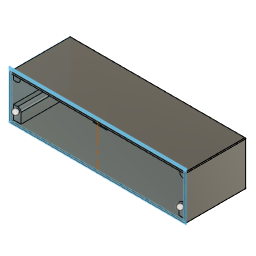
Midi Thru Box Enclosure v1 (Autodesk Fusion 360 design; units mm, degrees)
Autodesk Fusion 360 part; units mm, degrees
sketch "Sketch1" plane through (0, 0, 0) normal (0, 1, 0) x (1, 0, 0)
  line L0 (-3.1741, -17.9194) -> (125.8259, -17.9194) construction
  line L1 (125.8259, -17.9194) -> (125.8259, 15.0806) construction
  line L2 (125.8259, 15.0806) -> (-3.1741, 15.0806) construction
  line L3 (-3.1741, 15.0806) -> (-3.1741, -17.9194) construction
  circle A0 centre (-0.1741, 7.5806) radius 1.5 construction
  line L4 (61.3259, -17.9194) -> (61.3259, 15.0806)
  circle A1 centre (122.8259, 7.5806) radius 1.5 construction
  line L5 (-3.2741, -18.0194) -> (125.9259, -18.0194)
  line L6 (125.9259, -18.0194) -> (125.9259, 15.1806)
  line L7 (125.9259, 15.1806) -> (-3.2741, 15.1806)
  line L8 (-3.2741, 15.1806) -> (-3.2741, -18.0194)
  line L9 (-4.4741, -19.2194) -> (127.1259, -19.2194)
  line L10 (127.1259, -19.2194) -> (127.1259, 16.3806)
  line L11 (127.1259, 16.3806) -> (-4.4741, 16.3806)
  line L12 (-4.4741, 16.3806) -> (-4.4741, -19.2194)
  dimension "d1" = 129
  dimension "d2" = 33
  dimension "d6" = 3
  dimension "d7" = 6
  dimension "d8" = 1.5
  dimension "d11" = 0.1
  dimension "d12" = 1.3
  constraint horizontal L0
  constraint vertical L1
  constraint horizontal L2
  constraint vertical L3
  constraint midpoint L0 L4.start
  constraint midpoint L2 L4.end
  constraint symmetric A0 L4 A1
  measures "d1" distance of L0.start L0.end
  measures "d2" distance of L0.start L2.end
  measures "d6" diameter of A0
  measures "d7" distance of L2 A0
  measures "d8" distance of L3 A0
extrude "Extrude1" add sketch "Sketch1" along normal blind 44 makes body 1
sketch "Sketch2" plane through (0, 44, 0) normal (0, 1, 0) x (-1, 0, 0)
  line L0 (3.2741, 18.0194) -> (3.2741, -15.1806)
  line L1 (3.2741, -15.1806) -> (-125.9259, -15.1806)
  line L2 (-125.9259, -15.1806) -> (-125.9259, 18.0194)
  line L3 (-125.9259, 18.0194) -> (3.2741, 18.0194)
  line L4 (4.4741, -16.3806) -> (4.4741, 19.2194)
  line L5 (4.4741, 19.2194) -> (-127.1259, 19.2194)
  line L6 (-127.1259, 19.2194) -> (-127.1259, -16.3806)
  line L7 (-127.1259, -16.3806) -> (4.4741, -16.3806)
extrude "Extrude2" add sketch "Sketch2" along normal blind 1.2 contours L0 L1 L2 L3 | L4 L5 L6 L7 bodies 1
sketch "Sketch3" plane through (-3.2741, 0, 0) normal (1, 0, 0) x (0, 1, 0)
  line L0 (0, 18.0194) -> (0, -15.1806)
  line L1 (0, -15.1806) -> (44, -15.1806)
  line L2 (44, -15.1806) -> (44, 18.0194)
  line L3 (44, 18.0194) -> (0, 18.0194)
sketch "Sketch4" plane through (0, 44, 0) normal (0, -1, 0) x (1, 0, 0)
  line L0 (125.9259, 18.0194) -> (-3.2741, 18.0194)
  line L1 (-3.2741, 18.0194) -> (-3.2741, -15.1806)
  line L2 (-3.2741, -15.1806) -> (125.9259, -15.1806)
  line L3 (125.9259, -15.1806) -> (125.9259, 18.0194)
  line L4 (-3.2741, 18.0194) -> (1.7259, 18.0194)
  line L5 (1.7259, 18.0194) -> (1.7259, 15.5194)
  line L6 (-0.7741, 13.0194) -> (-3.2741, 13.0194)
  line L7 (-3.2741, 13.0194) -> (-3.2741, 18.0194)
  arc A0 (-0.7741, 13.0194) -> (1.7259, 15.5194) centre (-0.7741, 15.5194) ccw
  line L8 (61.3259, 18.0194) -> (61.3259, -15.1806)
  line L9 (-3.2741, 1.4194) -> (125.9259, 1.4194)
  line L10 (120.9259, 18.0194) -> (120.9259, 15.5194)
  line L11 (125.9259, 18.0194) -> (120.9259, 18.0194)
  line L12 (125.9259, 13.0194) -> (125.9259, 18.0194)
  line L13 (123.4259, 13.0194) -> (125.9259, 13.0194)
  arc A1 (120.9259, 15.5194) -> (123.4259, 13.0194) centre (123.4259, 15.5194) ccw
  line L14 (-3.2741, -15.1806) -> (2.7259, -15.1806)
  line L15 (-3.2741, -4.6806) -> (-3.2741, -15.1806)
  circle A2 centre (-0.1741, -7.5806) radius 1.5
  circle A3 centre (-0.1741, -7.5806) radius 1.3
  line L16 (-3.2741, -5.0806) -> (-0.1741, -5.0806)
  line L17 (2.3259, -7.5806) -> (2.3259, -15.1806)
  arc A4 (2.3259, -7.5806) -> (-0.1741, -5.0806) centre (-0.1741, -7.5806) ccw
  line L18 (61.3259, 17.9194) -> (61.3259, -15.0806)
  line L19 (125.9259, -5.0806) -> (122.8259, -5.0806)
  arc A5 (122.8259, -5.0806) -> (120.3259, -7.5806) centre (122.8259, -7.5806) ccw
  line L20 (120.3259, -7.5806) -> (120.3259, -15.1806)
  circle A6 centre (122.8259, -7.5806) radius 1.3
  dimension "d17" = 5
  dimension "d18" = 5
  dimension "d19" = 2.5
  dimension "d24" = 2.6
  dimension "d25" = 5
  constraint horizontal L4
  constraint vertical L5
  constraint horizontal L6
  constraint vertical L7
  constraint coincident L0.end L1.start
  constraint tangent L5 A0
  constraint tangent L6 A0
  constraint midpoint L0 L8.start
  constraint midpoint L2 L8.end
  constraint midpoint L1 L9.start
  constraint midpoint L3 L9.end
  constraint symmetric L0.end L8 L0.start
  constraint symmetric L4.end L8 L10.start
  constraint symmetric L6.end L8 L12.start
  constraint symmetric L5.end L8 L10.end
  constraint symmetric L6.start L8 L13.start
  constraint symmetric A0 L8 A1
  constraint horizontal L14
  constraint vertical L15
  constraint coincident L1.end L2.start
  constraint concentric A2 A3
  constraint concentric A3 A4
  constraint coincident L15 L16.start
  constraint horizontal L16
  constraint tangent L16 A4
  constraint coincident L2 L17.end
  constraint perpendicular L2 L17
  constraint tangent L17 A4
  constraint symmetric A3 L18 A6
  constraint symmetric L16.start L18 L19.start
  constraint symmetric L17.end L18 L20.end
  constraint symmetric L16.end L18 L19.end
  constraint symmetric L17.start L18 A5.end
  constraint symmetric A4 L18 A5
  measures "d17" distance of L0.end L4.end
  measures "d18" distance of L0.end L6.end
  measures "d19" radius of A0
  measures "d24" diameter of A3
  measures "d25" diameter of A4
extrude "Extrude3" add sketch "Sketch4" along normal blind 42.3 contours L0 L3 L10 L11 L12 L13 A1 | L0 L1 L4 L5 L6 L7 A0 | L2 L3 L19 A5 L20 | L1 L2 L14 L15 L16 L17 A4 | A2 | A3 | A6 bodies 1
sketch "Sketch5" plane through (0, 1.7, 0) normal (0, -1, 0) x (1, 0, 0)
  line L0 (-3.2741, -5.0806) -> (-3.2741, -15.1806)
  line L1 (-3.2741, -15.1806) -> (2.3259, -15.1806)
  line L2 (2.3259, -15.1806) -> (2.3259, -7.5806)
  arc A0 (2.3259, -7.5806) -> (-0.1741, -5.0806) centre (-0.1741, -7.5806) ccw
  line L3 (-0.1741, -5.0806) -> (-3.2741, -5.0806)
  circle A1 centre (-0.1741, -7.5806) radius 1.5
  circle A2 centre (-0.1741, -7.5806) radius 1.3
  circle A3 centre (122.8259, -7.5806) radius 1.5
  circle A4 centre (122.8259, -7.5806) radius 1.3
  dimension "d28" = 2.6
  dimension "d29" = 2.6
  constraint concentric A1 A2
  constraint concentric A3 A4
  measures "d28" diameter of A2
  measures "d29" diameter of A4
extrude "Extrude4" cut sketch "Sketch5" against normal blind 10 contours A2 | A4 bodies 1
sketch "Sketch6" plane through (0, 45.2, 0) normal (0, 1, 0) x (-1, 0, 0)
  line L0 (-127.1259, -16.3806) -> (4.4741, -16.3806)
  line L1 (4.4741, -16.3806) -> (4.4741, 19.2194)
  line L2 (4.4741, 19.2194) -> (-127.1259, 19.2194)
  line L3 (-127.1259, 19.2194) -> (-127.1259, -16.3806)
  line L4 (-125.9259, 18.0194) -> (-125.9259, -15.1806)
  line L5 (-125.9259, -15.1806) -> (3.2741, -15.1806)
  line L6 (-125.9259, -15.1806) -> (-116.4259, -15.1806)
  line L7 (-116.4259, -15.1806) -> (-85.4259, -15.1806)
  line L8 (-85.4259, -15.1806) -> (-76.4259, -15.1806)
  circle A0 centre (-79.9259, -2.6806) radius 3.5
  dimension "d32" = 9.5
  dimension "d33" = 31
  dimension "d34" = 9
  dimension "d35" = 7
  dimension "d36" = 9
  constraint coincident L4.end L5.start
  constraint perpendicular L4 L6
  constraint parallel L5 L7
  constraint parallel L5 L8
  measures "d32" distance of L4.end L6.end
  measures "d33" distance of L6.end L7.end
  measures "d34" distance of L7.end L8.end
  measures "d35" diameter of A0
  measures "d36" distance of L8 A0
extrude "Extrude6" cut sketch "Sketch6" against normal blind 30 contours A0 bodies 1
extrude "Extrude5" cut sketch "Sketch6" against normal blind 5 contours A0 bodies 1
fillet "Fillet1" radius 0.5 8 edges at (127.1259, 22.6, 19.2194) (-4.4741, 22.6, 19.2194) (61.3259, 45.2, 19.2194) (127.1259, 45.2, 1.4194) (127.1259, 22.6, -16.3806) (61.3259, 45.2, -16.3806) (-4.4741, 45.2, 1.4194) (-4.4741, 22.6, -16.3806) on bodies 1
fillet "Fillet2" radius 1 16 edges at (61.3259, 44, 18.0194) (1.7259, 44, 16.7694) (0.9937, 44, 13.7517) (-2.0241, 44, 13.0194) (-3.2741, 44, 3.9694) (124.6759, 44, 13.0194) (121.6581, 44, 13.7517) (120.9259, 44, 16.7694) (125.9259, 44, 3.9694) (120.3259, 44, -11.3806) (121.0581, 44, -5.8128) (124.3759, 44, -5.0806) (61.3259, 44, -15.1806) (-1.7241, 44, -5.0806) (1.5937, 44, -5.8128) (2.3259, 44, -11.3806) on bodies 1
sketch "Sketch7" plane through (127.1259, 0, 0) normal (1, 0, 0) x (0, 1, 0)
  line L0 (0, 18.7194) -> (0, -15.8806)
  line L1 (45.2, -15.8806) -> (45.2, 18.7194)
  line L2 (0, 19.2194) -> (0, -16.3806)
  line L3 (0, 5) -> (45.2, 5)
  line L4 (45.2, 5) -> (45.2, 2.5)
  line L5 (45.2, 2.5) -> (0, 2.5)
  line L6 (0, 2.5) -> (0, 5)
  dimension "d45" = 2.5
  constraint horizontal L3
  constraint vertical L4
  constraint horizontal L5
  constraint vertical L6
  constraint coincident L0 L3.start
  measures "d45" distance of L3.start L5.end
extrude "Extrude7" cut sketch "Sketch7" against normal blind 145 bodies 1 makes body 2 at (39.5592, 29.8, -16.3806)
move_body "Align1" bodies 1 to x (1, 0, 0) y (0, 1, 0) z (0, 0, 1) at (0, 0, -2.5)
combine "Combine1" operation add target body 1 tool bodies 2
ref_plane "WorkPlane1" through (61.3259, 22.35, 0.1694) normal (1, 0, 0) x (0, 0, -1)
sketch "Sketch8" plane through (61.3259, 22.35, 0.1694) normal (1, 0, 0) x (0, 1, 0)
  line L0 (20.65, 10.35) -> (20.65, 12.85)
  line L1 (20.65, 12.85) -> (-20.65, 12.85)
  line L2 (-20.65, 12.85) -> (-20.65, 10.35)
  line L3 (-20.65, 10.35) -> (20.65, 10.35)
  line L4 (20.65, 12.85) -> (20.65, 15.35)
  line L5 (20.65, 15.35) -> (-20.65, 15.35)
  line L6 (-20.65, 15.35) -> (-20.65, 12.85)
  line L7 (-20.65, 12.85) -> (20.65, 12.85)
  line L8 (-20.65, 15.35) -> (-20.65, 12.85)
  line L9 (-20.65, 15.35) -> (-0.65, 15.35)
  line L10 (-20.65, 12.85) -> (-0.65, 15.35)
  dimension "d48" = 20
  constraint coincident L5.end L6.start
  constraint coincident L1.end L2.start
  constraint perpendicular L8 L9
  measures "d48" distance of L5.end L9.end
extrude "Extrude9" add sketch "Sketch8" against normal blind 5 contours L5 L6 L8 L9 L10 bodies 1
extrude "Extrude8" add sketch "Sketch8" along normal blind 5 contours L5 L6 L8 L9 L10 bodies 1
